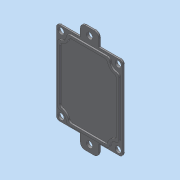
# Autodesk Inventor part: tapa
Saved by Autodesk Inventor 2013 (Build 170138000, 138)
## iProperties
Created: 2017-05-15
Part Number: tapa
Material: Generic
Document SubType Name: Modeling
Designer: Fede
Density: 1 g/cm^3
Author: Fede
Autodesk Inventor part; units mm, degrees
ref_plane "YZ Plane" through (0, 0, 0) normal (1, 0, 0) x (0, 1, 0)
ref_plane "XZ Plane" through (0, 0, 0) normal (0, 1, 0) x (-1, 0, 0)
ref_plane "XY Plane" through (0, 0, 0) normal (0, 0, 1) x (1, 0, 0)
sketch "Sketch1" plane through (0, 0, 0) normal (0, 1, 0) x (-1, 0, 0)
  line L0 (378.9658, -444.1109) -> (421.9658, -444.1109)
  line L1 (421.9658, -444.1109) -> (421.9658, -498.1109)
  line L2 (421.9658, -498.1109) -> (378.9658, -498.1109)
  line L3 (378.9658, -498.1109) -> (378.9658, -444.1109)
  point P0 (0, 0)
  dimension "d0" = 43
  dimension "d1" = 54
  constraints: 8 end point, 2 parallel, 1 horizontal, 1 perpendicular
  measures "d0" distance of L1.end L2.end
  measures "d1" distance of L0.end L1.end
extrude "Extrusion1" add sketch "Sketch1" along normal blind 1.6
sketch "Sketch2" plane through (-421.9658, 0, -444.1109) normal (0, 0, 1) x (1, 0, 0)
  line L0 (43, 0) -> (0, 0) projected
  line L1 (43, 0) -> (43, 1.6) projected
  line L2 (0, 1.6) -> (43, 1.6) projected
  line L3 (0, 0) -> (0, 1.6) projected
  line L4 (15.5, 1.6) -> (27.5, 1.6)
  line L5 (27.5, 1.6) -> (27.5, 0)
  line L6 (27.5, 0) -> (15.5, 0)
  line L7 (15.5, 0) -> (15.5, 1.6)
  point P0 (421.9658, 0)
  dimension "d4" = 15.5
  dimension "d5" = 15.5
  constraints: 8 end point, 2 parallel, 2 point on line, 1 horizontal, 1 perpendicular
  measures "d4" distance between parallel lines of L7 L3
  measures "d5" distance between parallel lines of L1 L5
sketch "Sketch3" plane through (-378.9658, 0, -498.1109) normal (0, 0, -1) x (-1, 0, 0)
  line L0 (43, 0) -> (0, 0) projected
  line L1 (43, 0) -> (43, 1.6) projected
  line L2 (0, 1.6) -> (43, 1.6) projected
  line L3 (0, 0) -> (0, 1.6) projected
  line L4 (15.5, 1.6) -> (27.5, 1.6)
  line L5 (27.5, 1.6) -> (27.5, 0)
  line L6 (27.5, 0) -> (15.5, 0)
  line L7 (15.5, 0) -> (15.5, 1.6)
  point P0 (-378.9658, 0)
  dimension "d6" = 15.5
  dimension "d7" = 15.5
  constraints: 8 end point, 2 parallel, 2 point on line, 1 horizontal, 1 perpendicular
  measures "d6" distance between parallel lines of L3 L7
  measures "d7" distance between parallel lines of L1 L5
extrude "Extrusion2" add sketch "Sketch2" along normal blind 8 contours L0 L7 L2 L5
extrude "Extrusion3" add sketch "Sketch3" along normal blind 8 contours L0 L7 L2 L5
sketch "Sketch4" plane through (0, 1.6, 0) normal (0, 1, 0) x (1, 0, 0)
  line L0 (-421.9658, 444.1109) -> (-406.4658, 444.1109) projected
  line L1 (-394.4658, 436.1109) -> (-406.4658, 436.1109) projected
  line L2 (-394.4658, 444.1109) -> (-378.9658, 444.1109) projected
  line L3 (-378.9658, 444.1109) -> (-378.9658, 498.1109) projected
  line L4 (-378.9658, 498.1109) -> (-394.4658, 498.1109) projected
  line L5 (-406.4658, 506.1109) -> (-394.4658, 506.1109) projected
  line L6 (-406.4658, 498.1109) -> (-421.9658, 498.1109) projected
  line L7 (-421.9658, 498.1109) -> (-421.9658, 444.1109) projected
  point P0 (0, 0)
  point P1 (-400.4658, 501.6109)
  point P2 (-400.4658, 440.6109)
  point P3 (-418.9658, 447.1109)
  point P4 (-418.9658, 495.1109)
  point P5 (-381.9658, 495.1109)
  point P6 (-381.9658, 447.1109)
  dimension "d12" = 3
  dimension "d13" = 3
  dimension "d14" = 3
  dimension "d15" = 3
  dimension "d16" = 3
  dimension "d17" = 3
  dimension "d18" = 3
  dimension "d19" = 3
  dimension "d20" = 4.5
  dimension "d21" = 4.5
  measures "d12" distance from line of L6 point (-418.966, 495.111)
  measures "d13" distance from line of L7 point (-418.966, 495.111)
  measures "d14" distance from line of L3 point (-381.966, 495.111)
  measures "d15" distance from line of point (-381.966, 495.111) L4
  measures "d16" distance from line of L2 point (-381.966, 447.111)
  measures "d17" distance from line of L3 point (-381.966, 447.111)
  measures "d18" distance from line of L0 point (-418.966, 447.111)
  measures "d19" distance from line of L7 point (-418.966, 447.111)
  measures "d20" distance from line of L5 point (-400.466, 501.611)
  measures "d21" distance from line of L1 point (-400.466, 440.611)
hole "Hole1" at (-400.4658, 1.6, -501.6109) at (-400.4658, 1.6, -440.6109) at (-418.9658, 1.6, -447.1109) at (-418.9658, 1.6, -495.1109) at (-381.9658, 1.6, -495.1109) at (-381.9658, 1.6, -447.1109) direction (0, -1, 0) diameter 4 end through all
chamfer "Chamfer1" distance 0.2 angle 45 4 edges at (-418.9658, 1.6, -449.1109) (-381.9658, 1.6, -449.1109) (-381.9658, 1.6, -497.1109) (-418.9658, 1.6, -497.1109)
fillet "Fillet1" radius 0.75 12 edges at (-414.2158, 1.6, -444.1109) (-406.4658, 1.6, -440.1109) (-400.4658, 1.6, -436.1109) (-394.4658, 1.6, -440.1109) (-378.9658, 1.6, -471.1109) (-386.7158, 1.6, -444.1109) (-386.7158, 1.6, -498.1109) (-394.4658, 1.6, -502.1109) (-400.4658, 1.6, -506.1109) (-406.4658, 1.6, -502.1109) (-414.2158, 1.6, -498.1109) (-421.9658, 1.6, -471.1109)
sketch "Sketch5" plane through (0, 0, 0) normal (0, -1, 0) x (1, 0, 0)
  circle A0 centre (-381.9658, -495.1109) radius 2 projected
  circle A1 centre (-418.9658, -447.1109) radius 2 projected
  circle A2 centre (-418.9658, -495.1109) radius 2 projected
  circle A3 centre (-381.9658, -447.1109) radius 2 projected
  line L0 (-406.4658, -444.1109) -> (-421.9658, -444.1109) projected
  line L1 (-421.9658, -444.1109) -> (-421.9658, -498.1109) projected
  line L2 (-394.4658, -498.1109) -> (-378.9658, -498.1109) projected
  line L3 (-378.9658, -498.1109) -> (-378.9658, -444.1109) projected
  line L4 (-412.5854, -445.6109) -> (-388.3463, -445.6109)
  line L5 (-380.4658, -453.4913) -> (-380.4658, -488.7304)
  line L6 (-388.3463, -496.6109) -> (-412.5854, -496.6109)
  line L7 (-420.4658, -488.7304) -> (-420.4658, -453.4913)
  line L8 (-389.6853, -495.0109) -> (-411.2464, -495.0109)
  line L9 (-382.0658, -454.8303) -> (-382.0658, -487.3914)
  arc A4 (-386.3524, -447.4546) -> (-382.3096, -451.4974) centre (-381.9658, -447.1109) ccw
  arc A5 (-382.3096, -490.7243) -> (-386.3524, -494.7671) centre (-381.9658, -495.1109) ccw
  arc A6 (-414.5793, -494.7671) -> (-418.6221, -490.7243) centre (-418.9658, -495.1109) ccw
  arc A7 (-413.1762, -493.5359) -> (-417.3908, -489.3213) centre (-418.9658, -495.1109) ccw
  arc A8 (-418.6221, -451.4974) -> (-414.5793, -447.4546) centre (-418.9658, -447.1109) ccw
  arc A9 (-417.3908, -452.9005) -> (-413.1762, -448.6859) centre (-418.9658, -447.1109) ccw
  arc A10 (-421.8586, -444.1109) -> (-421.9658, -444.2181) centre (-418.9658, -447.1109) ccw
  line L10 (-411.2464, -447.2109) -> (-389.6853, -447.2109)
  line L11 (-418.8658, -487.3914) -> (-418.8658, -454.8303)
  arc A11 (-387.7554, -448.6859) -> (-383.5408, -452.9005) centre (-381.9658, -447.1109) ccw
  arc A12 (-379.0043, -498.1109) -> (-378.9658, -498.0724) centre (-381.9658, -495.1109) ccw
  arc A13 (-383.5408, -489.3213) -> (-387.7554, -493.5359) centre (-381.9658, -495.1109) ccw
  arc A14 (-418.6221, -451.4974) -> (-420.4658, -453.4913) centre (-418.4658, -453.4913) ccw
  arc A15 (-417.3908, -452.9005) -> (-418.8658, -454.8303) centre (-416.8658, -454.8303) ccw
  arc A16 (-412.5854, -445.6109) -> (-414.5793, -447.4546) centre (-412.5854, -447.6109) ccw
  arc A17 (-411.2464, -447.2109) -> (-413.1762, -448.6859) centre (-411.2464, -449.2109) ccw
  arc A18 (-387.7554, -448.6859) -> (-389.6853, -447.2109) centre (-389.6853, -449.2109) ccw
  arc A19 (-386.3524, -447.4546) -> (-388.3463, -445.6109) centre (-388.3463, -447.6109) ccw
  arc A20 (-380.4658, -453.4913) -> (-382.3096, -451.4974) centre (-382.4658, -453.4913) ccw
  arc A21 (-382.0658, -454.8303) -> (-383.5408, -452.9005) centre (-384.0658, -454.8303) ccw
  arc A22 (-382.3096, -490.7243) -> (-380.4658, -488.7304) centre (-382.4658, -488.7304) ccw
  arc A23 (-383.5408, -489.3213) -> (-382.0658, -487.3914) centre (-384.0658, -487.3914) ccw
  arc A24 (-389.6853, -495.0109) -> (-387.7554, -493.5359) centre (-389.6853, -493.0109) ccw
  arc A25 (-388.3463, -496.6109) -> (-386.3524, -494.7671) centre (-388.3463, -494.6109) ccw
  arc A26 (-414.5793, -494.7671) -> (-412.5854, -496.6109) centre (-412.5854, -494.6109) ccw
  arc A27 (-413.1762, -493.5359) -> (-411.2464, -495.0109) centre (-411.2464, -493.0109) ccw
  arc A28 (-420.4658, -488.7304) -> (-418.6221, -490.7243) centre (-418.4658, -488.7304) ccw
  arc A29 (-418.8658, -487.3914) -> (-417.3908, -489.3213) centre (-416.8658, -487.3914) ccw
  point P0 (0, 0)
  point P1 (-414.8294, -445.6109)
  point P2 (-386.1023, -496.6109)
  point P3 (-386.1023, -445.6109)
  point P4 (-387.965, -495.0109)
  point P5 (-418.8658, -489.1117)
  point P6 (-418.8658, -453.11)
  point P7 (-412.9667, -447.2109)
  point P8 (-420.4658, -451.2473)
  point P9 (-382.0658, -453.11)
  point P10 (-380.4658, -451.2473)
  point P11 (-387.965, -447.2109)
  point P12 (-380.4658, -490.9745)
  point P13 (-382.0658, -489.1117)
  point P14 (-412.9667, -495.0109)
  point P15 (-420.4658, -490.9745)
  point P16 (-414.8294, -496.6109)
  dimension "d33" = 1.6
  dimension "d35" = 1.6
  dimension "d36" = 1.6
  dimension "d37" = 1.6
  dimension "d38" = 1.6
  dimension "d39" = 1.6
  dimension "d41" = 1.6
  dimension "d42" = 40
  dimension "d43" = 51
  dimension "d44" = 1.5
  dimension "d45" = 1.5
  dimension "d47" = 6
  dimension "d48" = 1.6
  dimension "d49" = 6
  dimension "d50" = 2
  constraints: 68 point on circle, 32 tangent, 26 centre point, 20 point on line, 17 equal radius, 16 end point, 4 coincident, 4 concentric, 4 parallel, 2 horizontal, 2 perpendicular
  measures "d33" distance between parallel lines of L4 L10
  measures "d35" distance between parallel lines of L5 L9
  measures "d36" distance between parallel lines of L6 L8
  measures "d37" distance between parallel lines of L11 L7
  measures "d38" radial gap between concentric circles of A9 A8
  measures "d39" radial gap between concentric circles of A4 A11
  measures "d41" radial gap between concentric circles of A7 A6
  measures "d42" distance between parallel lines of L5 L7
  measures "d43" distance between parallel lines of L6 L4
  measures "d44" distance between parallel lines of L1 L7
  measures "d45" distance between parallel lines of L2 L6
  measures "d47" radius of A7
  measures "d48" radial gap between concentric circles of A13 A5
  measures "d49" radius of A13
  measures "d50" radius of A14
extrude "Extrusion4" add sketch "Sketch5" along normal blind 1 contours L4 A19 A4 A20 L5 A22 A5 A25 L6 A26 A6 A28 L7 A14 A8 A16
fillet "Fillet2" radius 3 8 edges at (-406.2462, 1.3803, -436.3306) (-406.4658, 0.425, -436.1109) (-406.2462, 1.3803, -505.8912) (-406.4658, 0.425, -506.1109) (-394.6855, 1.3803, -436.3306) (-394.4658, 0.425, -436.1109) (-394.6855, 1.3803, -505.8912) (-394.4658, 0.425, -506.1109)
fillet "Fillet3" radius 2 8 edges at (-379.1855, 1.3803, -497.8912) (-378.9658, 0.425, -498.1109) (-379.1855, 1.3803, -444.3306) (-378.9658, 0.425, -444.1109) (-421.7462, 1.3803, -497.8912) (-421.9658, 0.425, -498.1109) (-421.7462, 1.3803, -444.3306) (-421.9658, 0.425, -444.1109)
body "Solid1"
